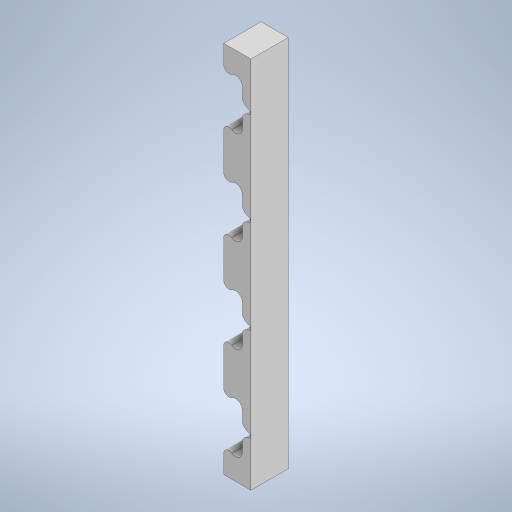
# Autodesk Inventor part: Zipperteeth
Saved by Autodesk Inventor 2023.1 (Build 271208000, 208)
## iProperties
Created: 2022-09-13
Part Number: Zipperteeth
Material: Generic
Document SubType Name: Modeling
Designer: Grimm
Density: 1 g/cm^3
Appearance: Default
Author: Grimm
Autodesk Inventor part; units mm, degrees
ref_plane "YZ Plane" through (0, 0, 0) normal (1, 0, 0) x (0, 1, 0)
ref_plane "XZ Plane" through (0, 0, 0) normal (0, 1, 0) x (-1, 0, 0)
ref_plane "XY Plane" through (0, 0, 0) normal (0, 0, 1) x (1, 0, 0)
sketch "Sketch1" plane through (0, 0, 0) normal (0, 0, 1) x (1, 0, 0)
  line L0 (-37.9485, 83.8136) -> (0.1515, 83.8136)
  line L1 (0.1515, 83.8136) -> (0.1515, -43.1864)
  line L2 (0.1515, -43.1864) -> (-37.9485, -43.1864)
  line L3 (-37.9485, -43.1864) -> (-37.9485, 83.8136)
  point P0 (0, 0)
  dimension "d0" = 38.1
  dimension "d1" = 127
  constraints: 8 end point, 2 parallel, 1 horizontal, 1 perpendicular
  measures "d0" distance of L1.end L2.end
  measures "d1" distance of L0.end L1.end
extrude "Extrusion1" add sketch "Sketch1" along normal blind 50.8
sketch "Sketch2" plane through (0, 0, 50.8) normal (0, 0, 1) x (1, 0, 0)
  line L0 (-12.5485, 45.1133) -> (-12.5485, -4.4861)
  arc A0 (-12.5485, 45.1133) -> (-25.2485, 52.0636) centre (-20.8003, 45.1133) ccw
  arc A1 (-37.9485, 59.0139) -> (-25.2485, 52.0636) centre (-29.6967, 59.0139) ccw
  arc A2 (-12.5485, 45.1133) -> (-25.2485, 52.0636) centre (-20.8003, 45.1133) ccw
  arc A3 (-37.9485, 59.0139) -> (-25.2485, 52.0636) centre (-29.6967, 59.0139) ccw
  arc A4 (-25.2485, -11.4364) -> (-12.5485, -4.4861) centre (-20.8003, -4.4861) ccw
  arc A5 (-25.2485, -11.4364) -> (-37.9485, -18.3867) centre (-29.6967, -18.3867) ccw
  line L1 (0.1515, -43.1864) -> (0.1515, 83.8136) projected
  line L2 (-37.9485, -43.1864) -> (0.1515, -43.1864) projected
  line L3 (0.1515, 83.8136) -> (-37.9485, 83.8136) projected
  line L4 (-37.9485, 83.8136) -> (-37.9485, -43.1864) projected
  line L5 (-29.6967, 59.0139) -> (-20.8003, 45.1133) construction
  line L6 (0.1515, 20.3136) -> (-4.9285, 20.3136)
  line L7 (-37.9485, 59.0139) -> (-37.9485, -18.3867)
  point P0 (0, 0)
  point P1 (0, 0)
  point P2 (-12.5485, 20.3136)
  dimension "d32" = 63.5
  dimension "d34" = 25.4
  dimension "d35" = 5.08
  constraints: 12 point on circle, 8 end point, 7 tangent, 6 centre point, 4 equal radius, 3 point on line, 2 midpoint, 2 vertical alignment, 1 collinear, 1 horizontal, 1 horizontal alignment, 1 vertical
  measures "d32" distance of A4.start A0.end
  measures "d34" distance between parallel lines of L4 L0
  measures "d35" distance of L6.start L6.end
extrude "Extrusion2" cut sketch "Sketch2" against normal through all contours L0 A4 A5 L4 A1 A0
thicken "Thicken1" operation cut thickness 1 both sides no extend neighbours no toward (1, 0, 0) faces at (-37.9485, 75.547, 16.9333) (-33.3682, 51.6239, 16.9333) (-16.5551, 52.1894, 16.9333) (-12.5485, 12.047, 33.8667) (-22.8599, -12.4768, 16.9333) (-37.845, -17.084, 16.9333) (-37.9485, -34.9198, 33.8667)
sketch "Sketch4" plane through (0, 0, 50.8) normal (0, 0, 1) x (1, 0, 0)
  line L0 (-0.6485, 22.8136) -> (-0.6485, 17.8136)
  line L1 (-12.5485, 45.1133) -> (-12.5485, -4.4861) projected
  line L2 (-12.5485, 20.3136) -> (0.1515, 20.3136) construction
  line L3 (0.1515, -43.1864) -> (0.1515, 83.8136) projected
  arc A0 (-12.5485, 34.7136) -> (-0.6485, 22.8136) centre (0.1278, 35.4898) ccw
  line L4 (-0.6485, 22.8136) -> (-12.5485, 34.7136) construction
  line L5 (-0.6485, 22.8136) -> (16.1807, 22.8136) construction
  arc A1 (-0.6485, 17.8136) -> (-12.5485, 5.9136) centre (0.1278, 5.1373) ccw
  line L6 (-0.6485, 17.8136) -> (-12.5485, 5.9136) construction
  line L7 (-0.6485, 17.8136) -> (16.1807, 17.8136) construction
  point P0 (0, 0)
  point P1 (-0.6485, 20.3136)
  dimension "d41" = 5
  dimension "d42" = 0.8
  constraints: 12 end point, 4 point on circle, 3 midpoint, 3 point on line, 2 centre point, 2 equal length, 2 horizontal, 1 vertical
  measures "d41" distance of L0.start L0.end
  measures "d42" distance between parallel lines of L3 L0
extrude "Extrusion4" cut sketch "Sketch4" against normal through all
pattern_linear "Rectangular Pattern1" count 4 spacing 127 along (0, 1, 0)
body "Solid1"
